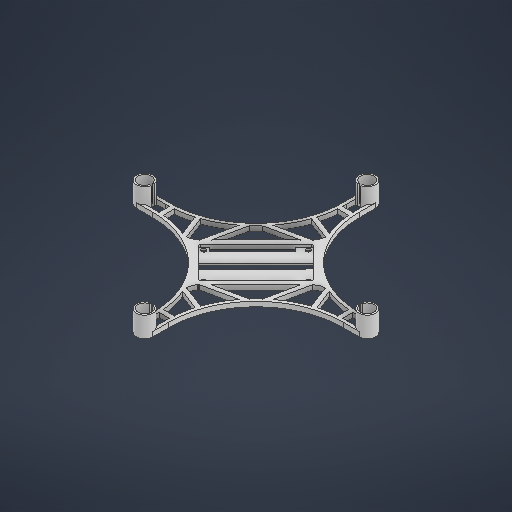
# Autodesk Inventor part: Part1
Saved by Autodesk Inventor 2026.1 (Build 301233020, 233B)
## iProperties
Created: 2025-12-23
Part Number: Part1
Material: Generic
Document SubType Name: Modeling
Designer: ferrm
Density: 1 g/cm^3
Appearance: Default
Author: ferrm
Autodesk Inventor part; units mm, degrees
ref_plane "YZ Plane" through (0, 0, 0) normal (1, 0, 0) x (0, 1, 0)
ref_plane "XZ Plane" through (0, 0, 0) normal (0, 1, 0) x (-1, 0, 0)
ref_plane "XY Plane" through (0, 0, 0) normal (0, 0, 1) x (1, 0, 0)
sketch "Sketch1" plane through (0, 0, 0) normal (0, 1, 0) x (-1, 0, 0)
  circle A0 centre (70.75, 0) radius 4
  circle A1 centre (70.75, 0) radius 5.25
  circle A2 centre (0, 70.75) radius 4
  circle A3 centre (0, 70.75) radius 5.25
  circle A4 centre (-70.75, 0) radius 4
  circle A5 centre (-70.75, 0) radius 5.25
  circle A6 centre (0, -70.75) radius 4
  circle A7 centre (0, -70.75) radius 5.25
  line L0 (70.75, -5.25) -> (60.75, -5.25)
  line L1 (5.25, -70.75) -> (5.25, -60.75)
  arc A8 (60.75, -5.25) -> (5.25, -60.75) centre (60.75, -60.75) ccw
  line L2 (5.25, 70.75) -> (5.25, 60.75)
  arc A9 (5.25, 60.75) -> (60.75, 5.25) centre (60.75, 60.75) ccw
  line L3 (70.75, 5.25) -> (60.75, 5.25)
  line L4 (-70.75, 5.25) -> (-60.75, 5.25)
  arc A10 (-60.75, 5.25) -> (-5.25, 60.75) centre (-60.75, 60.75) ccw
  line L5 (-5.25, 70.75) -> (-5.25, 60.75)
  line L6 (-5.25, -70.75) -> (-5.25, -60.75)
  arc A11 (-5.25, -60.75) -> (-60.75, -5.25) centre (-60.75, -60.75) ccw
  line L7 (-70.75, -5.25) -> (-60.75, -5.25)
  line L8 (3.25, -66.6269) -> (3.25, -60.75)
  arc A12 (60.75, -3.25) -> (3.25, -60.75) centre (60.75, -60.75) ccw
  line L9 (60.75, -3.25) -> (66.6269, -3.25)
  line L10 (3.25, 60.75) -> (3.25, 66.6269)
  arc A13 (3.25, 60.75) -> (60.75, 3.25) centre (60.75, 60.75) ccw
  line L11 (66.6269, 3.25) -> (60.75, 3.25)
  line L12 (-60.75, 3.25) -> (-66.6269, 3.25)
  arc A14 (-60.75, 3.25) -> (-3.25, 60.75) centre (-60.75, 60.75) ccw
  line L13 (-3.25, 66.6269) -> (-3.25, 60.75)
  line L14 (-3.25, -60.75) -> (-3.25, -66.6269)
  arc A15 (-3.25, -60.75) -> (-60.75, -3.25) centre (-60.75, -60.75) ccw
  line L15 (-66.6269, -3.25) -> (-60.75, -3.25)
  line L16 (8.6716, 30.5919) -> (30.5919, 8.6716)
  line L17 (-30.1824, -8.2621) -> (-8.2621, -30.1824)
  line L18 (5.8432, 30.5919) -> (-30.1824, -5.4337)
  line L19 (30.5919, 5.8432) -> (-5.4337, -30.1824)
  arc A16 (30.5919, 5.8432) -> (30.5919, 8.6716) centre (29.1777, 7.2574) ccw
  arc A17 (8.6716, 30.5919) -> (5.8432, 30.5919) centre (7.2574, 29.1777) ccw
  arc A18 (-30.1824, -5.4337) -> (-30.1824, -8.2621) centre (-28.7682, -6.8479) ccw
  arc A19 (-8.2621, -30.1824) -> (-5.4337, -30.1824) centre (-6.8479, -28.7682) ccw
  line L20 (27.5771, 8.8388) -> (8.8388, 27.5771)
  line L21 (27.5771, 7.4246) -> (-7.4246, -27.5772)
  line L22 (7.4246, 27.5771) -> (-27.5772, -7.4246)
  line L23 (-27.5772, -8.8389) -> (-8.8389, -27.5772)
  arc A20 (8.8388, 27.5771) -> (7.4246, 27.5771) centre (8.1317, 26.87) ccw
  arc A21 (-27.5772, -7.4246) -> (-27.5772, -8.8389) centre (-26.8701, -8.1317) ccw
  arc A22 (-8.8389, -27.5772) -> (-7.4246, -27.5772) centre (-8.1317, -26.8701) ccw
  arc A23 (27.5771, 7.4246) -> (27.5771, 8.8388) centre (26.87, 8.1317) ccw
  arc A24 (-38.8996, -7.5634) -> (-30.1824, -5.4337) centre (-36.2945, 0.6784) ccw
  arc A25 (38.8996, 7.5634) -> (30.1824, 5.4337) centre (36.2945, -0.6784) ccw
  arc A26 (-5.8914, -30.5246) -> (-7.4296, -39.2282) centre (0.303, -36.1071) ccw
  arc A27 (38.8996, 7.5634) -> (30.1824, 5.4337) centre (36.2945, -0.6784) ccw
  arc A28 (5.8914, 30.5246) -> (7.4296, 39.2282) centre (-0.303, 36.1071) ccw
  line L24 (58.3526, -3.3) -> (58.3526, 3.3)
  line L25 (55.3939, -3.5) -> (55.3939, 3.5)
  line L26 (3.3, 58.3526) -> (-3.3, 58.3526)
  line L27 (3.5, 55.3939) -> (-3.5, 55.3939)
  line L28 (-58.3526, 3.3) -> (-58.3526, -3.3)
  line L29 (-55.3939, 3.5) -> (-55.3939, -3.5)
  line L30 (-3.3, -58.3526) -> (3.3, -58.3526)
  line L31 (-3.5, -55.3939) -> (3.5, -55.3939)
  point P0 (0, 0)
  point P1 (-3.4781, -55.6334)
  point P2 (5.1659, -46.0308)
  point P3 (28.2843, 8.1317)
  point P4 (8.1317, 28.2843)
  point P5 (-8.1317, -28.2843)
  point P6 (70.75, 5.25)
  point P7 (-5.25, 70.75)
  point P8 (-70.75, 5.25)
  point P9 (-70.75, -5.25)
  point P10 (-5.25, -70.75)
  point P11 (-3.25, -66.6269)
  point P12 (66.6269, 3.25)
  point P13 (-66.6269, -3.25)
  point P14 (-3.25, 66.6269)
  point P15 (3.25, 66.6269)
  point P16 (38.8996, 7.5634)
  point P17 (7.4296, 39.2282)
  point P18 (6.1802, 30.8628)
  dimension "d1" = 8
  dimension "d2" = 70.75
  dimension "d3" = 10.5
  dimension "d6" = 360
  dimension "d8" = 10
  dimension "d9" = 10
  dimension "d12" = 360
  dimension "d14" = 2
  dimension "d17" = 360
  dimension "d23" = 35
  dimension "d24" = 17.5
  dimension "d25" = 2
  dimension "d28" = 28.5
  dimension "d29" = 51.5
  dimension "d30" = 3.25
  dimension "d31" = 2.0135
  dimension "d32" = 1
  dimension "d45" = 360
  dimension "d47" = 8.6438
  dimension "d50" = 135
  dimension "d54" = 54.9478
  dimension "d55" = 27.7635
  dimension "d56" = 2
  dimension "d58" = 0
  dimension "d60" = 67.5
  dimension "d66" = 63.3769
  dimension "d68" = 63.3769
  dimension "d70" = 69.8769
  dimension "d74" = 67.5
  dimension "d76" = 74
  dimension "d92" = 0
  dimension "d94" = 6.5
  dimension "d96" = 2
  dimension "d98" = 8.5
  dimension "d102" = 360
  dimension "d104" = 8.3387
  dimension "d105" = 35.9782
  dimension "d106" = 7
  dimension "d107" = 6.6
  dimension "d110" = 360
  constraints: 64 end point, 55 point on circle, 29 centre point, 24 tangent, 6 equal radius, 6 point on line, 4 coincident, 4 perpendicular, 3 parallel, 3 vertical, 1 horizontal, 134 other
  measures "d1" diameter of A0
  measures "d2" distance of point (0, 0) A0.centre
  measures "d3" diameter of A1
  measures "d8" distance of L0.start L0.end
  measures "d9" distance of L1.start L1.end
  measures "d14" radial gap between concentric circles of A8 A12
  measures "d23" distance between parallel lines of L18 L19
  measures "d24" distance from line of L18 point (0, 0)
  measures "d25" radius of A16
  measures "d28" distance of point (28.284, 8.132) point (8.132, 28.284)
  measures "d29" distance of point (28.284, 8.132) point (-8.132, -28.284)
  measures "d30" distance between parallel lines of L22 L18
  measures "d31" distance between parallel lines of L20 L16
  measures "d32" radius of A20
  measures "d47" radius of A25
  measures "d50" angle of L11 L16
  measures "d54" distance between parallel lines of L17 L16
  measures "d55" distance from line of point (0, 0) L16
  measures "d56" distance from line of point (70.75, 5.25) L11
  measures "d58" distance from line of point (66.627, 3.25) L11
  measures "d60" distance from line of point (5.25, 70.75) L11
  measures "d66" distance from line of point (3.25, 66.627) L11
  measures "d68" distance from line of point (-3.25, 66.627) L11
  measures "d70" distance from line of point (-3.25, -66.627) L11
  measures "d74" distance from line of point (-5.25, 70.75) L11
  measures "d76" distance from line of point (-5.25, -70.75) L11
  measures "d92" distance from line of point (-66.627, 3.25) L11
  measures "d94" distance from line of point (-66.627, -3.25) L11
  measures "d96" distance from line of point (-70.75, 5.25) L11
  measures "d98" distance from line of point (-70.75, -5.25) L11
  measures "d104" radius of A26
  measures "d105" distance from line of A28.end L11
  measures "d106" distance of L25.start L25.end
  measures "d107" distance of L24.start L24.end
extrude "Extrusion1" add sketch "Sketch1" along normal blind 3 contours A1 | A1 L11 A13 L10 A3 L2 A9 L3 | L0 A8 L1 A7 L8 A12 L9 A1 | L24 A12 L25 A13 | A3 | A7 | A3 L13 A14 L12 A5 L4 A10 L5 | L6 A11 L7 A5 L15 A15 L14 A7 | A25 L19 A16 L16 A17 A28 A13 | A12 L30 A15 L31 | L19 A19 L17 A18 L18 A17 L16 A16 | A13 L27 A14 L26 | A5 | A15 A24 A18 L17 A19 A26 | L29 A15 L28 A14
sketch "Sketch2" plane through (0, 0, 0) normal (0, -1, 0) x (1, 0, 0)
  line L0 (-27.5771, 7.4246) -> (7.4246, -27.5772) projected
  arc A0 (7.4246, -27.5772) -> (8.8389, -27.5772) centre (8.1317, -26.8701) ccw projected
  line L1 (8.8389, -27.5772) -> (27.5772, -8.8389) projected
  arc A1 (27.5772, -8.8389) -> (27.5772, -7.4246) centre (26.8701, -8.1317) ccw projected
  line L2 (27.5772, -7.4246) -> (-7.4246, 27.5771) projected
  line L3 (-8.8388, 27.5771) -> (-27.5771, 8.8388) projected
  arc A2 (-27.5771, 8.8388) -> (-27.5771, 7.4246) centre (-26.87, 8.1317) ccw projected
  arc A3 (-7.4246, 27.5771) -> (-8.8388, 27.5771) centre (-8.1317, 26.87) ccw projected
  point P0 (0, 0)
extrude "Extrusion2" add sketch "Sketch2" against normal blind 1.2
sketch "Sketch3" plane through (0, 1.2, 0) normal (0, 1, 0) x (1, 0, 0)
  arc A0 (27.5772, 7.4246) -> (27.5772, 8.8389) centre (26.8701, 8.1317) ccw projected
  line L0 (27.5772, 8.8389) -> (26.7287, 9.6874)
  line L1 (8.8389, 27.5772) -> (27.5772, 8.8389) projected
  line L2 (27.5772, 7.4246) -> (26.7287, 6.5761)
  line L3 (27.5772, 7.4246) -> (-7.4246, -27.5771) projected
  line L4 (26.7287, 9.6874) -> (25.173, 8.1317)
  line L5 (25.173, 8.1317) -> (26.7287, 6.5761)
  line L6 (-25.173, -8.1317) -> (-26.7287, -6.5761)
  line L7 (-26.7287, -9.6874) -> (-25.173, -8.1317)
  line L8 (-27.5771, -7.4246) -> (7.4246, 27.5772) projected
  line L9 (7.4246, 27.5772) -> (8.9803, 26.0215)
  line L10 (8.9803, 26.0215) -> (8.1317, 25.173)
  line L11 (-7.4246, -27.5772) -> (-8.9803, -26.0215)
  line L12 (-8.9803, -26.0215) -> (-8.1317, -25.173)
  point P0 (0, 0)
  dimension "d114" = 1.2
  dimension "d115" = 1.2
  dimension "d118" = 360
  dimension "d122" = 2.2
  dimension "d123" = 1.2
  dimension "d126" = 360
  constraints: 20 end point, 2 point on line, 22 other
  measures "d114" distance of L0.start L0.end
  measures "d115" distance of L2.start L2.end
  measures "d122" distance of L8.end L9.end
  measures "d123" distance of L9.end L10.end
hole "Hole1" at (25.173, 1.2, -8.1317) at (8.1317, 1.2, -25.173) at (-8.1317, 1.2, 25.173) at (-25.173, 1.2, 8.1317) direction (0, -1, 0) diameter 3 end through all
sketch "Sketch4" plane through (0, 1.2, 0) normal (0, 1, 0) x (1, 0, 0)
  circle A0 centre (25.173, 8.1317) radius 1.5 projected
  circle A1 centre (-8.1317, -25.173) radius 1.5 projected
  line L0 (5.6213, 22.663) -> (-22.663, -5.6212)
  line L1 (5.6213, 22.663) -> (4.0659, 24.2184)
  line L2 (-27.5771, -7.4246) -> (7.4246, 27.5772) projected
  line L3 (-22.663, -5.6212) -> (-24.2184, -4.0658)
  line L4 (4.0659, 24.2184) -> (-24.2184, -4.0658)
  line L5 (24.2184, 4.0659) -> (-4.0658, -24.2184)
  line L6 (27.5772, 7.4246) -> (-7.4246, -27.5771) projected
  line L7 (8.8389, 27.5772) -> (27.5772, 8.8389) projected
  line L8 (18.208, 18.208) -> (-18.208, -18.208)
  line L9 (-8.8388, -27.5771) -> (-27.5771, -8.8388) projected
  line L10 (22.663, 5.6213) -> (-5.6212, -22.663)
  line L11 (22.663, 5.6213) -> (24.2184, 4.0659)
  line L12 (-5.6212, -22.663) -> (-4.0658, -24.2184)
  point P0 (0, 0)
  point P1 (25.668, 5.5155)
  point P2 (-5.5155, -25.668)
  dimension "d138" = 40
  dimension "d139" = 5.75
  constraints: 18 end point, 4 symmetric about line, 2 collinear, 2 midpoint, 2 point on line, 1 perpendicular
  measures "d138" distance between parallel lines of L3 L1
  measures "d139" distance between parallel lines of L7 L1
extrude "Extrusion3" cut sketch "Sketch4" against normal up to surface (1.2 mm away) contours L0 L3 L2 L1 | L5 L12 L10 L11
sketch "Sketch6" plane through (0, 3, 0) normal (0, 1, 0) x (1, 0, 0)
  line L0 (0, 70.722) -> (-3.9999, 70.722)
  circle A0 centre (0, 70.75) radius 4 projected
  line L1 (-70.722, 0) -> (-70.722, -3.9999)
  line L2 (0, -70.722) -> (3.9999, -70.722)
  line L3 (70.722, 0) -> (70.722, 3.9999)
  point P0 (0, 0)
  dimension "d143" = 360
  constraints: 8 end point, 1 horizontal, 15 other
hole "Hole2" at (0, 3, -70.722) at (-70.722, 3, 0) at (0, 3, 70.722) at (70.722, 3, 0) direction (0, -1, 0) diameter 8.5 end through all
sketch "Sketch7" plane through (0, 0, 0) normal (0, -1, 0) x (1, 0, 0)
  circle A0 centre (0, -70.722) radius 4.25 projected
  circle A1 centre (0, -70.722) radius 3.4
  circle A2 centre (70.722, 0) radius 3.4
  circle A3 centre (0, 70.722) radius 3.4
  circle A4 centre (-70.722, 0) radius 3.4
  circle A5 centre (0, -70.722) radius 4.25
  circle A6 centre (70.722, 0) radius 4.25
  circle A7 centre (0, 70.722) radius 4.25
  circle A8 centre (-70.722, 0) radius 4.25
  point P0 (0, 0)
  dimension "d152" = 6.8
  dimension "d155" = 360
  dimension "d159" = 360
  constraints: 8 centre point, 2 coincident, 1 concentric, 18 other
  measures "d152" diameter of A1
extrude "Extrusion4" add sketch "Sketch7" against normal blind 1.2
sketch "Sketch8" plane through (0, 0, 0) normal (0, -1, 0) x (1, 0, 0)
  circle A0 centre (70.722, 0) radius 3.4 projected
  line L0 (67.5049, 1.1) -> (67.5049, -1.1)
  line L1 (67.5049, 1.1) -> (65.6165, 1.1)
  arc A1 (66.6269, 3.25) -> (66.6269, -3.25) centre (70.75, 0) ccw projected
  line L2 (67.5049, -1.1) -> (65.6165, -1.1)
  arc A2 (67.5049, 1.1) -> (67.5049, -1.1) centre (70.722, 0) ccw
  arc A3 (65.6165, 1.1) -> (65.6165, -1.1) centre (70.75, 0) ccw
  line L3 (-1.1, 67.5049) -> (-1.1, 65.6165)
  arc A4 (-1.1, 67.5049) -> (1.1, 67.5049) centre (0, 70.722) ccw
  line L4 (1.1, 67.5049) -> (1.1, 65.6165)
  arc A5 (-1.1, 65.6165) -> (1.1, 65.6165) centre (0, 70.75) ccw
  line L5 (-67.5049, -1.1) -> (-65.6165, -1.1)
  arc A6 (-67.5049, -1.1) -> (-67.5049, 1.1) centre (-70.722, 0) ccw
  line L6 (-67.5049, 1.1) -> (-65.6165, 1.1)
  arc A7 (-65.6165, -1.1) -> (-65.6165, 1.1) centre (-70.75, 0) ccw
  line L7 (1.1, -67.5049) -> (1.1, -65.6165)
  arc A8 (1.1, -67.5049) -> (-1.1, -67.5049) centre (0, -70.722) ccw
  line L8 (-1.1, -67.5049) -> (-1.1, -65.6165)
  arc A9 (1.1, -65.6165) -> (-1.1, -65.6165) centre (0, -70.75) ccw
  point P0 (0, 0)
  dimension "d163" = 2.2
  dimension "d166" = 360
  constraints: 20 point on circle, 18 end point, 8 centre point, 1 concentric, 1 horizontal, 1 vertical, 41 other
  measures "d163" distance of L0.start L0.end
extrude "Extrusion5" cut sketch "Sketch8" against normal through all contours A0 L2 A1 L1 | A4 L4 A5 L3 | A6 L6 A7 L5 | A8 L8 A9 L7
sketch "Sketch10" plane through (0, 0, 0) normal (0, -1, 0) x (1, 0, 0)
  line L0 (-1.5059, 13.9748) -> (13.9554, -1.6761)
  line L1 (13.9554, -1.6761) -> (1.6252, -14.0944)
  line L2 (1.6252, -14.0944) -> (-14.1071, 1.5262)
  line L3 (-14.1071, 1.5262) -> (-1.5059, 13.9748)
  line L4 (-1.5059, 13.9748) -> (-2.9569, 15.4437)
  line L5 (-0.1134, -12.3682) -> (1.6128, -10.6296)
  line L6 (3.3514, -12.3558) -> (1.6128, -10.6296)
  circle A0 centre (1.6128, -10.6296) radius 1.75
  line L7 (12.09, 0.2122) -> (10.1835, -1.6713)
  line L8 (12.0853, -3.5596) -> (10.1835, -1.6713)
  circle A1 centre (10.1835, -1.6713) radius 1.75
  line L9 (-1.5059, 13.9748) -> (-2.3843, 14.864)
  line L10 (-15.8834, 1.5285) -> (1.6315, -15.8622)
  line L11 (1.6315, -15.8622) -> (15.7147, -1.6783)
  line L12 (15.7147, -1.6783) -> (-1.4951, 15.7425)
  line L13 (-1.4951, 15.7425) -> (-15.8834, 1.5285)
  line L14 (-1.5059, 13.9748) -> (-2.3843, 14.864)
  line L15 (-1.5059, 13.9748) -> (-0.6166, 14.8533)
  line L16 (-14.1071, 1.5262) -> (-14.9878, 0.6392)
  point P0 (0, 0)
  dimension "d170" = 22
  dimension "d171" = 17.5
  dimension "d172" = 8.75
  dimension "d173" = 11
  dimension "d177" = 2.45
  dimension "d178" = 2.45
  dimension "d179" = 3.5
  dimension "d186" = 2.68
  dimension "d187" = 2.68
  dimension "d188" = 3.5
  dimension "d202" = 1.25
  constraints: 34 end point, 10 perpendicular, 7 point on line, 2 centre point, 2 coincident, 1 collinear, 3 other
  measures "d170" distance of L0.start L0.end
  measures "d171" distance of L0.end L1.end
  measures "d172" distance from line of point (0, 0) L0
  measures "d173" distance from line of L3 point (0, 0)
  measures "d177" distance of L5.end L5.start
  measures "d178" distance of L6.start L5.end
  measures "d179" diameter of A0
  measures "d186" distance of L7.start L7.end
  measures "d187" distance of L7.end L8.start
  measures "d188" diameter of A1
  measures "d202" distance between parallel lines of L2 L10
extrude "Extrusion6" cut sketch "Sketch10" against normal through all contours L15 L12 L11 L10 L16 L2 L1 L0 | A1 L8 L7 | L7 L8 A1
sketch "Sketch11" plane through (0, 3, 0) normal (0, 1, 0) x (1, 0, 0)
  arc A0 (1.1, 66.6168) -> (-1.1, 66.6168) centre (0, 70.722) ccw projected
  circle A1 centre (0, 70.722) radius 4.25
  arc A2 (5.25, 70.75) -> (-5.25, 70.75) centre (0, 70.75) ccw projected
  circle A3 centre (0, 70.75) radius 5.25
  line L0 (-1.1, 65.6165) -> (-1.1, 66.6168) projected
  line L1 (-1.1, 66.6168) -> (-1.1, 65.6165)
  line L2 (1.1, 66.6168) -> (1.1, 65.6165)
  circle A4 centre (-70.722, 0) radius 4.25
  circle A5 centre (-70.75, 0) radius 5.25
  line L3 (-66.6168, 1.1) -> (-65.6165, 1.1)
  line L4 (-66.6168, -1.1) -> (-65.6165, -1.1)
  circle A6 centre (0, -70.722) radius 4.25
  circle A7 centre (0, -70.75) radius 5.25
  line L5 (-1.1, -66.6168) -> (-1.1, -65.6165)
  line L6 (1.1, -66.6168) -> (1.1, -65.6165)
  circle A8 centre (70.722, 0) radius 4.25
  circle A9 centre (70.75, 0) radius 5.25
  line L7 (66.6168, -1.1) -> (65.6165, -1.1)
  line L8 (66.6168, 1.1) -> (65.6165, 1.1)
  point P0 (0, 0)
  dimension "d182" = 360
  constraints: 16 end point, 8 centre point, 4 point on circle, 2 coincident, 2 vertical, 41 other
extrude "Extrusion7" add sketch "Sketch11" along normal blind 10 contours A0 L0 A3 A2 L2 | A4 L4 A5 L3 | A6 L6 A7 L5 | A8 L8 A9 L7 picked at (-75.5648, 0.7599) picked at (4.8247, -71.4981) picked at (75.5648, -0.7599)
sketch "Sketch12" plane through (0, 0, 0) normal (0, -1, 0) x (1, 0, 0)
  arc A0 (-3.5, -55.3939) -> (-55.3939, -3.5) centre (-60.75, -60.75) ccw projected
  line L0 (5.4337, -30.1824) -> (-30.1824, 5.4337) projected
  line L1 (-30.1824, 5.4337) -> (-25.7867, -15.1011)
  line L2 (5.4337, -30.1824) -> (-15.1011, -25.7867)
  line L3 (1.7678, -26.5165) -> (-18.0126, -22.2823)
  line L4 (-26.513, 1.7642) -> (-22.2789, -18.0157)
  line L5 (0, 0) -> (-21.5056, 21.5056)
  arc A1 (-60.75, 5.25) -> (-5.25, 60.75) centre (-60.75, 60.75) ccw projected
  line L6 (-5.4337, 30.1824) -> (15.1011, 25.7867)
  line L7 (30.1824, -5.4337) -> (25.7867, 15.1011)
  line L8 (26.5165, -1.7678) -> (22.2823, 18.0126)
  line L9 (-1.7642, 26.513) -> (18.0157, 22.2789)
  arc A2 (3.5, 55.3939) -> (55.3939, 3.5) centre (60.75, 60.75) ccw projected
  line L10 (-5.8432, 30.5919) -> (30.1824, -5.4337) projected
  point P0 (5.8914, -30.5246)
  dimension "d189" = 21
  dimension "d190" = 20.2284
  dimension "d191" = 21
  dimension "d192" = 20.228
  constraints: 18 end point, 8 symmetric about line, 5 point on circle, 3 parallel, 2 point on line
  measures "d189" distance of L0.start L2.end
  measures "d190" distance of L3.start L3.end
  measures "d191" distance of L0.end L1.end
  measures "d192" distance of L4.start L4.end
extrude "Extrusion8" add sketch "Sketch12" against normal up to surface (3 mm away) contours A0 L3 L0 L2 | A0 L1 L0 L4 | L6 A2 L9 L10 | L8 A2 L7 L10
sketch "Sketch13" plane through (0, 1.2, 0) normal (0, 1, 0) x (1, 0, 0)
  line L0 (-22.663, -5.6212) -> (5.6213, 22.663) projected
  line L1 (5.6213, 22.663) -> (6.1516, 22.1327)
  line L2 (-22.663, -5.6212) -> (-22.1327, -6.1516)
  line L3 (6.1516, 22.1327) -> (-22.1327, -6.1516)
  line L4 (-24.2184, -4.0658) -> (-22.663, -5.6212) projected
  line L5 (5.6213, 22.663) -> (-22.663, -5.6212)
  line L6 (-5.6212, -22.663) -> (22.663, 5.6213) projected
  line L7 (-5.6212, -22.663) -> (-6.1516, -22.1327)
  line L8 (22.663, 5.6213) -> (22.1327, 6.1516)
  line L9 (22.1327, 6.1516) -> (-6.1516, -22.1327)
  line L10 (-5.6212, -22.663) -> (22.663, 5.6213)
  point P0 (0, 0)
  point P1 (-22.1327, -6.1516)
  dimension "d195" = 0.75
  dimension "d196" = 0.75
  dimension "d197" = 0.75
  dimension "d198" = 0.75
  constraints: 16 end point, 3 perpendicular, 2 equal length
  measures "d195" distance of L0.end L1.end
  measures "d196" distance of L0.start L2.end
  measures "d197" distance of L6.end L8.end
  measures "d198" distance of L6.start L7.end
extrude "Extrusion9" cut sketch "Sketch13" against normal through all
sketch "Sketch14" plane through (0, 1.2, 0) normal (0, 1, 0) x (1, 0, 0)
  line L0 (6.1516, 22.1327) -> (-22.1327, -6.1516) projected
  line L1 (-22.1327, -6.1516) -> (-22.8398, -6.8587)
  line L2 (-27.5771, -7.4246) -> (7.4246, 27.5772) projected
  line L3 (-22.8398, -6.8587) -> (-24.9255, -4.773)
  line L4 (-24.2184, -4.0658) -> (-24.9255, -4.773)
  line L5 (-24.2184, -4.0658) -> (-22.1327, -6.1516)
  line L6 (0, 0) -> (18.208, 18.208)
  line L7 (8.8389, 27.5772) -> (27.5772, 8.8389) projected
  line L8 (-6.1516, -22.1327) -> (-6.8587, -22.8398)
  line L9 (-7.4246, -27.5771) -> (27.5772, 7.4246)
  line L10 (-6.8587, -22.8398) -> (-4.773, -24.9255)
  line L11 (-4.0658, -24.2184) -> (-6.1516, -22.1327)
  dimension "d203" = 1
  constraints: 18 end point, 6 symmetric about line, 4 point on line, 2 perpendicular, 1 collinear, 1 midpoint
  measures "d203" distance of L0.end L1.end
extrude "Extrusion10" cut sketch "Sketch14" against normal through all
sketch "Sketch15" plane through (0, 1.2, 0) normal (0, 1, 0) x (1, 0, 0)
  line L0 (8.8389, 27.5772) -> (27.5772, 8.8389) projected
  line L1 (6.1516, 22.1327) -> (4.5606, 20.5417)
  line L2 (6.1516, 22.1327) -> (-22.8398, -6.8587) projected
  line L3 (4.5606, 20.5417) -> (2.4749, 22.6274)
  line L4 (-27.5771, -7.4246) -> (7.4246, 27.5772) projected
  line L5 (6.1516, 22.1327) -> (4.0659, 24.2184) projected
  line L6 (4.0659, 24.2184) -> (2.4749, 22.6274)
  line L7 (4.0659, 24.2184) -> (6.1516, 22.1327)
  line L8 (0, 0) -> (18.208, 18.208)
  line L9 (22.1327, 6.1516) -> (20.5417, 4.5606)
  line L10 (20.5417, 4.5606) -> (22.6274, 2.4749)
  line L11 (-7.4246, -27.5771) -> (27.5772, 7.4246)
  line L12 (22.1327, 6.1516) -> (24.2184, 4.0659)
  dimension "d206" = 2.25
  constraints: 18 end point, 6 symmetric about line, 3 point on line, 2 perpendicular, 1 collinear, 1 midpoint
  measures "d206" distance of L1.start L1.end
extrude "Extrusion11" add sketch "Sketch15" against normal up to surface (1.2 mm away)
sketch "Sketch16" plane through (0, 1.2, 0) normal (0, 1, 0) x (1, 0, 0)
  line L0 (-14.9878, -0.6392) -> (1.6315, 15.8622) projected
  line L1 (-14.9878, -0.6392) -> (-14.1071, -1.5262) projected
  line L2 (-14.9878, -0.6392) -> (-14.1071, -1.5262)
  line L3 (-14.1071, -1.5262) -> (1.5994, 14.0688)
  line L4 (13.9554, 1.6761) -> (-1.5059, -13.9748) projected
  line L5 (1.5994, 14.0688) -> (13.9554, 1.6761)
  line L6 (13.9554, 1.6761) -> (-1.5059, -13.9748)
  line L7 (-0.6166, -14.8533) -> (15.7147, 1.6783) projected
  line L8 (-1.5059, -13.9748) -> (-0.6166, -14.8533)
  line L9 (-0.6166, -14.8533) -> (15.7147, 1.6783)
  line L10 (15.7147, 1.6783) -> (1.6315, 15.8622)
  line L11 (-14.9878, -0.6392) -> (-14.1071, -1.5262)
  point P0 (0, 0)
  point P1 (-1.5059, -13.9748)
  constraints: 16 end point, 4 perpendicular, 1 collinear, 1 parallel
extrude "Extrusion12" add sketch "Sketch16" against normal up to surface (1.2 mm away)
sketch "Sketch17" plane through (0, 0, 0) normal (0, -1, 0) x (1, 0, 0)
  circle A0 centre (10.1835, -1.6713) radius 1.75 projected
  circle A1 centre (10.1835, -1.6713) radius 1.75
  point P0 (0, 0)
  constraints: 1 centre point, 1 coincident
extrude "Extrusion13" add sketch "Sketch17" against normal up to surface (1.2 mm away)
sketch "Sketch18" plane through (0, 1.2, 0) normal (0, 1, 0) x (1, 0, 0)
  line L0 (8.8389, 27.5772) -> (27.5772, 8.8389) projected
  line L1 (20.0428, 16.3732) -> (16.8637, 19.5523)
  line L2 (16.8637, 19.5523) -> (-19.5523, -16.8637)
  line L3 (-8.8388, -27.5771) -> (-27.5771, -8.8388) projected
  line L4 (20.0428, 16.3732) -> (-15.9975, -20.4185)
  line L5 (-19.5523, -16.8637) -> (-15.9975, -20.4185)
  line L6 (20.0428, 16.3732) -> (16.8637, 19.5523)
  point P0 (0, 0)
  constraints: 10 end point, 4 point on line, 1 collinear, 1 perpendicular
extrude "Extrusion14" cut sketch "Sketch18" against normal blind 10
sketch "Sketch19" plane through (0, 0, 0) normal (0, -1, 0) x (1, 0, 0)
  arc A0 (7.4296, -39.2282) -> (3.5, -55.3939) centre (60.75, -60.75) ccw projected
  line L0 (7.4296, -39.2282) -> (-5.6361, -44.3576)
  arc A1 (-3.5, -55.3939) -> (-15.1011, -25.7867) centre (-60.75, -60.75) ccw projected
  arc A2 (7.4296, -39.2282) -> (5.8914, -30.5246) centre (-0.303, -36.1071) ccw projected
  line L1 (8.0357, -36.1071) -> (-6.5034, -41.6829)
  line L2 (-8.0357, 36.1071) -> (6.5034, 41.6829)
  line L3 (-7.4296, 39.2282) -> (5.6361, 44.3576)
  arc A3 (30.1824, -5.4337) -> (38.8996, -7.5634) centre (36.2945, 0.6784) ccw projected
  arc A4 (25.7867, 15.1011) -> (55.3939, 3.5) centre (60.75, 60.75) ccw projected
  line L4 (0, 0) -> (8.0357, -36.1071)
  line L5 (0, 0) -> (0.2589, -1.1633)
  line L6 (41.683, 6.5033) -> (36.1237, -7.9637)
  arc A5 (55.3939, -3.5) -> (38.8996, -7.5634) centre (60.75, -60.75) ccw projected
  line L7 (44.3574, 5.6362) -> (39.2291, -7.4293)
  line L8 (-44.3574, -5.6362) -> (-39.2291, 7.4293)
  line L9 (-41.683, -6.5033) -> (-36.1237, 7.9637)
  arc A6 (3.5, 55.3939) -> (15.1011, 25.7867) centre (60.75, 60.75) ccw projected
  arc A7 (-7.4296, 39.2282) -> (-6.1802, 30.8628) centre (0.303, 36.1071) ccw projected
  arc A8 (-25.7867, -15.1011) -> (-55.3939, -3.5) centre (-60.75, -60.75) ccw projected
  arc A9 (-30.1824, 5.4337) -> (-38.8996, 7.5634) centre (-36.2945, -0.6784) ccw projected
  arc A10 (-55.3939, 3.5) -> (-38.8996, 7.5634) centre (-60.75, 60.75) ccw projected
  dimension "d217" = 360
  dimension "d222" = 36.9905
  dimension "d225" = 360
  dimension "d227" = 0.41
  dimension "d228" = 33.977
  dimension "d229" = 132.864
  dimension "d230" = 132.412
  dimension "d231" = 78.4627
  dimension "d232" = 73.1527
  dimension "d233" = 38.5654
  constraints: 20 end point, 7 point on circle, 1 point on line, 26 other
  measures "d222" distance of L4.start L1.start
  measures "d227" angle of L7 L6
  measures "d228" angle of L4 L7
  measures "d229" angle of L7 L0
  measures "d230" angle of L7 L1
  measures "d231" distance between parallel lines of L8 L7
  measures "d232" distance between parallel lines of L9 L6
  measures "d233" distance from line of L5.end L7
extrude "Extrusion15" add sketch "Sketch19" against normal blind 3 contours L0 A1 L1 A2 | A7 L3 A6 L2 | L6 A4 L7 A5 A3 | L8 A10 A9 L9 A8
body "Solid1"
